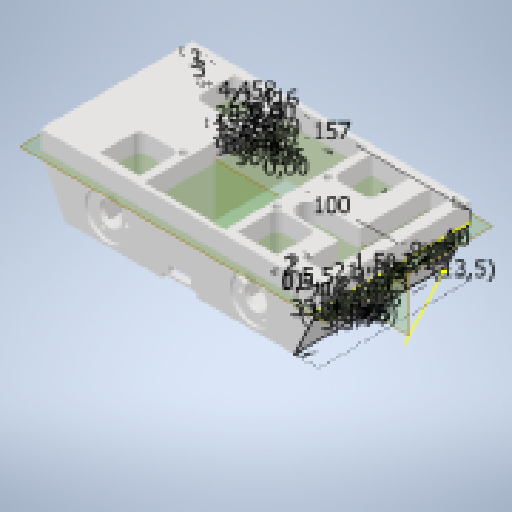
# Autodesk Inventor part: low_part
Saved by Autodesk Inventor 2025 (Build 290162000, 162)
## iProperties
Created: 2026-06-26
Part Number: low_part
Material: Типовые
Document SubType Name: Sheet Metal
Designer: garin
Density: 1 g/cm^3
Appearance: По умолчанию
Sheet Metal Rule: По умолчанию
Mass: 239.505 g
Surface Area: 434.405 cm^2
Volume: 239.505 cm^3
Author: garin
Autodesk Inventor part; units mm, degrees
ref_plane "YZ Plane" through (0, 0, 0) normal (1, 0, 0) x (0, 1, 0)
ref_plane "XZ Plane" through (0, 0, 0) normal (0, 1, 0) x (-1, 0, 0)
ref_plane "XY Plane" through (0, 0, 0) normal (0, 0, 1) x (1, 0, 0)
sketch "Эскиз2" plane through (0, 0, 0) normal (0, 0, 1) x (1, 0, 0)
  line L0 (0, 0) -> (-78.5, 0) construction
  line L1 (-78.5, 0) -> (78.5, 0)
  line L2 (0, 0) -> (-50, 0) construction
  line L3 (-50, 0) -> (-50, -28.5) construction
  line L4 (-50, -28.5) -> (-78.5, 0)
  line L5 (-50, -28.5) -> (50, -28.5)
  line L6 (50, -28.5) -> (78.5, 0)
  line L7 (-50, -28.5) -> (-45.542, -28.5) construction
  line L8 (-45.542, -28.5) -> (-45.542, -22.152) construction
  line L9 (-45.542, -22.152) -> (-50, -22.152) construction
  line L10 (-50, -22.152) -> (-50, -28.5) construction
  line L11 (-45.542, -22.152) -> (-45.542, -6.564) construction
  arc A0 (-45.542, -22.152) -> (-45.542, -6.564) centre (-50.0424, -14.358) ccw construction
  circle A1 centre (-45.542, -22.152) radius 1.3
  line L12 (-45.542, -22.152) -> (-32.0424, -14.358) construction
  line L13 (-45.542, -22.152) -> (-29.954, -22.152) construction
  circle A2 centre (-32.0424, -14.358) radius 1.3
  circle A3 centre (-45.542, -6.564) radius 1.3
  line L14 (-45.542, -6.564) -> (-32.0424, -14.358) construction
  circle A4 centre (-41.0424, -14.358) radius 12.5
  circle A5 centre (-41.0424, -14.358) radius 6.5
  line L15 (-41.0424, -14.358) -> (-41.0424, -26.858) construction
  line L16 (-41.0424, -14.358) -> (-34.7924, -25.1833) construction
  line L17 (-41.0424, -14.358) -> (-30.2171, -20.608) construction
  line L18 (-78.5, 0) -> (-75.5, 0) construction
  line L19 (-50, -28.5) -> (-47, -28.5) construction
  line L20 (-75.5, 0) -> (-47, -28.5)
  line L21 (-78.5, 0) -> (-75.5, 0) construction
  line L22 (-75.5, 0) -> (-75.5, -3) construction
  line L23 (-75.5, -3) -> (-78.5, -3) construction
  line L24 (-78.5, -3) -> (-78.5, 0) construction
  line L25 (-50, -28.5) -> (-50, -25.5) construction
  line L26 (-50, -28.5) -> (-47, -28.5) construction
  line L27 (-75.5, -3) -> (75.5, -3)
  line L28 (-75.5, -3) -> (75.5, -3) construction
  line L29 (0, 0) -> (0, -28.5) construction
  line L30 (75.5, 0) -> (47, -28.5)
  line L31 (-50, -25.5) -> (50, -25.5)
  line L32 (-50, -25.5) -> (50, -25.5) construction
  circle A6 centre (45.542, -22.152) radius 1.3
  circle A7 centre (32.0424, -14.358) radius 1.3
  circle A8 centre (45.542, -6.564) radius 1.3
  circle A9 centre (41.0424, -14.358) radius 12.5
  circle A10 centre (41.0424, -14.358) radius 6.5
  line L33 (41.0424, -14.358) -> (41.0424, -26.858) construction
  line L34 (41.0424, -14.358) -> (30.2171, -20.608) construction
  line L35 (-41.0424, -14.358) -> (-22.0786, -14.358) construction
  line L36 (-41.0424, -14.358) -> (-41.0424, -1.858)
  line L37 (-41.0424, -14.358) -> (-30.2171, -8.108)
  line L38 (41.0424, -14.358) -> (30.2171, -8.108)
  line L39 (41.0424, -14.358) -> (41.0424, -1.858)
  line L40 (-45.542, -6.564) -> (-50, -6.564) construction
  line L41 (-50, -6.564) -> (-50, 0) construction
  line L42 (-50, 0) -> (-45.542, 0) construction
  line L43 (-45.542, 0) -> (-45.542, -6.564) construction
  line L44 (-50, -25.5) -> (-27.584, -25.5)
  line L45 (-27.584, -25.5) -> (-27.584, 0)
  line L46 (-27.584, 0) -> (-50, 0)
  line L47 (-50, 0) -> (-50, -25.5)
  line L48 (27.584, -25.5) -> (27.584, 0)
  line L49 (50, 0) -> (50, -25.5)
  line L50 (-50, -28.5) -> (-65, -28.5)
  line L51 (-65, -28.5) -> (-78.5, 0)
  line L52 (-65, -28.5) -> (-62, -28.5)
  line L53 (-62, -28.5) -> (-75.5, 0)
  line L54 (-50, -25.5) -> (-63.4211, -25.5)
  line L55 (50, -28.5) -> (65, -28.5)
  line L56 (65, -28.5) -> (78.5, 0)
  line L57 (65, -28.5) -> (62, -28.5)
  line L58 (62, -28.5) -> (75.5, 0)
  point P0 (-72.5, -3)
  point P1 (72.5, -3)
  point P2 (-41.0424, -25.5)
  point P3 (-41.0424, -20.858)
  point P4 (-35.4132, -17.608)
  point P5 (-30.2171, -20.608)
  point P6 (-35.3762, -25.5)
  point P7 (35.3762, -25.5)
  point P8 (30.2171, -20.608)
  point P9 (35.4132, -17.608)
  point P10 (41.0424, -20.858)
  point P11 (41.0424, -25.5)
  point P12 (47, -28.5)
  point P13 (46.7086, -25.5)
  point P14 (41.0424, -26.858)
  point P15 (-46.7086, -25.5)
  point P16 (35.8226, -3)
  point P17 (41.0424, -3)
  point P18 (41.0424, -7.858)
  point P19 (35.4132, -11.108)
  point P20 (30.2171, -8.108)
  point P21 (-35.8226, -3)
  point P22 (-30.2171, -8.108)
  point P23 (-35.4132, -11.108)
  point P24 (-41.0424, -7.858)
  point P25 (-41.0424, -3)
  dimension "d0" = 78.5
  dimension "d1" = 157
  dimension "d2" = 50
  dimension "d3" = 28.5
  dimension "d4" = 100
  dimension "d15" = 4.458
  dimension "d16" = 6.348
  dimension "d17" = 15.588
  dimension "d18" = 9
  dimension "d19" = 2.6
  dimension "d20" = 15.588
  dimension "d21" = 30
  dimension "d22" = 2.6
  dimension "d23" = 2.6
  dimension "d24" = 25
  dimension "d25" = 13
  dimension "d26" = 12.5
  dimension "d29" = 30
  dimension "d31" = 3
  dimension "d32" = 3
  dimension "d33" = 3
  dimension "d34" = 90
  dimension "d35" = 0
  dimension "d36" = 0
  dimension "d48" = 4.458
  dimension "d49" = 22.416
  dimension "d151" = 15
  dimension "d152" = 3
  dimension "d153" = 15
  dimension "d154" = 3
  constraints: 118 end point, 17 symmetric about line, 13 point on line, 12 horizontal, 11 centre point, 9 parallel, 6 coincident, 5 perpendicular, 4 equal length, 3 point on circle, 3 vertical, 1 midpoint, 9 other
  measures "d0" distance of L0.start L0.end
  measures "d1" distance of L0.end L1.end
  measures "d2" distance of L0.start L2.end
  measures "d3" distance of L2.end L3.end
  measures "d4" distance of L3.end L5.end
  measures "d15" distance of L9.end L8.end
  measures "d16" distance of L8.end L7.end
  measures "d17" distance of L8.end L11.end
  measures "d18" radius of A0
  measures "d19" diameter of A1
  measures "d20" distance of L12.start L12.end
  measures "d21" angle of L13 L12
  measures "d22" diameter of A2
  measures "d23" diameter of A3
  measures "d24" diameter of A4
  measures "d25" diameter of A5
  measures "d26" distance of L15.start L15.end
  measures "d31" distance of L0.end L18.end
  measures "d32" distance of L3.end L19.end
  measures "d33" distance of L21.end L22.end
  measures "d34" angle of L26 L25
  measures "d35" distance between parallel lines of L27 L28
  measures "d36" distance between parallel lines of L31 L32
  measures "d48" distance of L41.end L42.end
  measures "d49" distance of L46.end L45.end
  measures "d151" distance of L3.end L50.end
  measures "d152" distance of L50.end L52.end
  measures "d153" distance of L5.end L55.end
  measures "d154" distance of L55.end L57.end
extrude "Выдавливание1" add sketch "Эскиз2" along normal blind 86 contours L1 L53 L27 L4 | L4 L53 L50 L51 | L1 L47 L27 L20 | L20 L27 L53 | L27 L53 L4 | L1 L45 L27 A4 L47 | L27 L47 A4 L20 | L20 L54 L4 L53 L27 | L4 L54 L53 | L53 L54 L4 L50 | L1 L48 L27 L45 | L27 A4 L47 | L31 A4 A9 L30 L5 L20 | L47 A4 L31 | L20 L5 L4 L54 | L1 L49 L27 A9 L48 | L45 L31 A4 L27 | L27 L48 L31 L45 | L27 L36 A5 L37 A4 L31 L47 | A4 L36 L27 | L47 A4 | L31 A4 | L1 L30 L27 L49 | L27 A9 L31 L48 | L27 L36 A4 | A4 L37 A5 L36 L27 | L30 L27 L58 L6 L5 | L58 L27 L30 | L1 L6 L27 L58 | L49 A9 L27 | L27 L30 L49 A9 | A9 L39 L27 | L27 L39 A10 L38 A9 | L36 L37 A5 | A5 L37 L36 | L6 L58 L55 | L31 A9 L49 | L56 L55 L58 L6 | L27 L6 L58 | A9 L49 L31 L38 A10 L39 L27 | L27 L39 A9 | A9 L49 | L31 A9 | L39 L38 A10 | A10 L38 L39 | A1 | A2 | A3 | A6 | A7 | A8
extrude "Выдавливание2" cut sketch "Эскиз2" along normal blind 5 contours A4 L37 A5 L36 L27 | L27 L39 A10 L38 A9 | L36 L37 A5 | A5 L37 L36 | L39 L38 A10 | A10 L38 L39 | A1 | A2 | A3 | A6 | A7 | A8
extrude "Выдавливание4" cut sketch "Эскиз2" along normal blind 2 contours L27 L36 A5 L37 A4 L31 L47 | A4 L36 L27 | L47 A4 | L31 A4 | L27 L36 A4 | A4 L37 A5 L36 L27 | A9 L39 L27 | L27 L39 A10 L38 A9 | L36 L37 A5 | A5 L37 L36 | A9 L49 L31 L38 A10 L39 L27 | L27 L39 A9 | A9 L49 | L31 A9 | L39 L38 A10 | A10 L38 L39 | A1 | A2 | A3 | A6 | A7 | A8
fillet "Сопряжение1" radius 2 4 edges at (35.4132, -11.108, 3.5) (41.0424, -7.858, 3.5) (-35.4132, -11.108, 3.5) (-41.0424, -7.858, 3.5)
extrude "Выдавливание6" cut sketch "Эскиз2" along normal blind 22.5 from surface at 5 contours L1 L45 L27 A4 L47 | L27 A4 L47 | L47 A4 L31 | L1 L49 L27 A9 L48 | L45 L31 A4 L27 | L27 L36 A5 L37 A4 L31 L47 | A4 L36 L27 | L27 A9 L31 L48 | L27 L36 A4 | A4 L37 A5 L36 L27 | L49 A9 L27 | A9 L39 L27 | L27 L39 A10 L38 A9 | L36 L37 A5 | A5 L37 L36 | L31 A9 L49 | A9 L49 L31 L38 A10 L39 L27 | L27 L39 A9 | L39 L38 A10 | A10 L38 L39 | A1 | A2 | A3 | A6 | A7 | A8
fillet "Сопряжение2" radius 4 4 edges at (50, -12.75, 27.5) (27.584, -12.75, 27.5) (-27.584, -12.75, 27.5) (-50, -12.75, 27.5)
ref_plane "РабПлоскость1" through (0, 0, 43) normal (0, 0, -1) x (-1, 0, 0)
mirror "Зеркальное отражение2" about plane through (0, 0, 43) normal (0, 0, -1) of "Выдавливание2", "Выдавливание6", "Сопряжение2", "Выдавливание4", "Сопряжение1"
sketch "Эскиз4" plane through (-78.5, 0, 0) normal (0, 1, 0) x (1, 0, 0)
  line L0 (78.5, 0) -> (78.5, -86) construction
  line L1 (28.5, -86) -> (128.5, -86) projected
  line L2 (0, 0) -> (0, -86) projected
  line L3 (0, -43) -> (157, -43) construction
  line L4 (157, 0) -> (157, -86) projected
  line L5 (78.5, -43) -> (101.4, -43) construction
  line L6 (101.4, -43) -> (101.4, -3) construction
  line L7 (101.4, -3) -> (78.5, -3) construction
  line L8 (78.5, -3) -> (78.5, -43) construction
  line L9 (101.4, -3) -> (55.6, -3)
  line L10 (55.6, -3) -> (55.6, -83)
  line L11 (55.6, -83) -> (101.4, -83)
  line L12 (101.4, -83) -> (101.4, -3)
  dimension "d53" = 22.9
  dimension "d54" = 40
  dimension "d55" = 45.8
  dimension "d56" = 80
  constraints: 20 end point, 4 midpoint, 4 parallel, 2 horizontal, 2 perpendicular
  measures "d53" distance of L7.end L6.end
  measures "d54" distance of L6.end L5.end
  measures "d55" distance of L11.end L10.end
  measures "d56" distance of L10.end L9.end
extrude "Выдавливание7" cut sketch "Эскиз4" against normal blind 28.5
sketch "Эскиз5" plane through (-78.5, 0, 0) normal (0, 1, 0) x (1, 0, 0)
  line L0 (0, 0) -> (157, 0)
  line L1 (157, 0) -> (157, -86)
  line L2 (157, -86) -> (0, -86)
  line L3 (0, -86) -> (0, 0)
  line L4 (55.6, -3) -> (101.4, -3) projected
  line L5 (55.6, -3) -> (55.6, -83) projected
  line L6 (101.4, -3) -> (55.6, -3)
  line L7 (55.6, -3) -> (55.6, -83)
  line L8 (55.6, -83) -> (101.4, -83)
  line L9 (101.4, -83) -> (101.4, -3)
  line L10 (104.4, 0) -> (52.6, 0)
  line L11 (52.6, 0) -> (52.6, -86)
  line L12 (52.6, -86) -> (104.4, -86)
  line L13 (104.4, -86) -> (104.4, 0)
  line L14 (3, -83) -> (154, -83)
  line L15 (154, -83) -> (154, -3)
  line L16 (154, -3) -> (3, -3)
  line L17 (3, -3) -> (3, -83)
  line L18 (104.4, 0) -> (106.084, 0)
  line L19 (106.084, 0) -> (106.084, -86)
  line L20 (106.084, -86) -> (104.4, -86)
  line L21 (104.4, -86) -> (104.4, 0)
  line L22 (52.6, 0) -> (50.916, 0)
  line L23 (50.916, 0) -> (50.916, -86)
  line L24 (50.916, -86) -> (52.6, -86)
  line L25 (52.6, -86) -> (52.6, 0)
  line L26 (50.916, 0) -> (52.916, 0) construction
  line L27 (0, -43) -> (157, -43) construction
  line L28 (78.5, -86) -> (78.5, 0) construction
  arc A0 (28.5, -23.5) -> (32.5, -27.5) centre (32.5, -23.5) ccw projected
  line L29 (46.916, -27.5) -> (32.5, -27.5) projected
  arc A1 (46.916, -27.5) -> (50.916, -23.5) centre (46.916, -23.5) ccw projected
  line L30 (50.916, -5) -> (50.916, -23.5) projected
  line L31 (50.916, -5) -> (28.5, -5) projected
  line L32 (28.5, -5) -> (28.5, -23.5) projected
  arc A2 (32.5, -58.5) -> (28.5, -62.5) centre (32.5, -62.5) ccw projected
  line L33 (28.5, -81) -> (28.5, -62.5) projected
  line L34 (50.916, -81) -> (28.5, -81) projected
  line L35 (50.916, -81) -> (50.916, -62.5) projected
  arc A3 (50.916, -62.5) -> (46.916, -58.5) centre (46.916, -62.5) ccw projected
  line L36 (46.916, -58.5) -> (32.5, -58.5) projected
  arc A4 (110.084, -58.5) -> (106.084, -62.5) centre (110.084, -62.5) ccw projected
  line L37 (106.084, -81) -> (106.084, -62.5) projected
  line L38 (128.5, -81) -> (106.084, -81) projected
  line L39 (128.5, -81) -> (128.5, -62.5) projected
  arc A5 (128.5, -62.5) -> (124.5, -58.5) centre (124.5, -62.5) ccw projected
  line L40 (124.5, -58.5) -> (110.084, -58.5) projected
  arc A6 (106.084, -23.5) -> (110.084, -27.5) centre (110.084, -23.5) ccw projected
  line L41 (124.5, -27.5) -> (110.084, -27.5) projected
  arc A7 (124.5, -27.5) -> (128.5, -23.5) centre (124.5, -23.5) ccw projected
  line L42 (128.5, -5) -> (128.5, -23.5) projected
  line L43 (128.5, -5) -> (106.084, -5) projected
  line L44 (106.084, -5) -> (106.084, -23.5) projected
  line L45 (46.916, -58.5) -> (55.6, -58.5) construction
  arc A8 (50.916, -62.5) -> (46.916, -58.5) centre (46.916, -62.5) ccw construction
  line L46 (46.916, -27.5) -> (55.6, -27.5) construction
  line L47 (55.6, -58.5) -> (52.1, -58.5) construction
  line L48 (52.1, -58.5) -> (52.1, -57.5) construction
  line L49 (52.1, -57.5) -> (55.6, -57.5) construction
  line L50 (55.6, -57.5) -> (55.6, -58.5) construction
  circle A9 centre (52.1, -57.5) radius 2.1
  circle A10 centre (52.1, -28.5) radius 2.1
  circle A11 centre (104.9, -57.5) radius 2.1
  circle A12 centre (104.9, -28.5) radius 2.1
  point P0 (50.916, -23.5)
  dimension "d59" = 157
  dimension "d60" = 86
  dimension "d61" = 3
  dimension "d62" = 3
  dimension "d63" = 1.684
  dimension "d64" = 1.684
  dimension "d72" = 3.5
  dimension "d73" = 1
  dimension "d74" = 4.2
  constraints: 66 end point, 14 parallel, 9 perpendicular, 6 horizontal, 4 centre point, 4 point on line, 3 midpoint, 3 symmetric about line, 3 tangent, 1 coincident, 1 vertical, 9 other
  measures "d59" distance of L1.end L2.end
  measures "d60" distance of L0.end L1.end
  measures "d61" distance between parallel lines of L9 L13
  measures "d62" distance between parallel lines of L2 L14
  measures "d63" distance of L19.end L20.end
  measures "d64" distance of L24.end L23.end
  measures "d72" distance of L48.end L49.end
  measures "d73" distance of L47.end L48.end
  measures "d74" diameter of A9
extrude "Выдавливание8" add sketch "Эскиз5" along normal blind 10.2 contours L0 L23 L16 L17 L14 L2 L3 | L0 L11 L16 L23 | L0 L13 L16 L4 L11 | L23 L31 L32 A0 L29 A1 A10 A9 A3 L36 A2 L33 L34 L14 L17 L16 | L16 L11 A10 L23 | L23 L14 L11 L2 | L0 L19 L16 L13 | L16 L5 L14 L11 A9 A10 | L11 L14 L8 L13 L2 | L23 A9 L11 L14 | L0 L1 L2 L19 L14 L15 L16 | L16 L19 A12 L13 | L13 A12 A11 L14 L9 L16 | L13 L14 L19 L2 | L16 L15 L14 L19 L38 L39 A5 L40 A4 A11 A12 A6 L41 A7 L42 L43 | L11 A9 L23 A10 | L13 A11 L19 L14 | A12 L19 A11 L13
sketch "Эскиз9" plane through (-65, -28.5, 0) normal (0, -1, 0) x (1, 0, 0)
  line L0 (130, 86) -> (143.5, 86) construction
  line L1 (0, 0) -> (130, 0) projected
  line L2 (143.5, 86) -> (130, 86) construction
  line L3 (130, 86) -> (130, 0) construction
  line L4 (130, 0) -> (143.5, 0) construction
  line L5 (143.5, 0) -> (143.5, 86) construction
  line L6 (130, 43) -> (87.9, 43) construction
  line L7 (87.9, 83) -> (87.9, 3) construction
  line L8 (130, 43) -> (87.9, 43) construction
  line L9 (87.9, 43) -> (87.9, 45) construction
  line L10 (87.9, 45) -> (130, 45) construction
  line L11 (130, 45) -> (130, 43) construction
  line L12 (130, 43) -> (87.9, 43) construction
  line L13 (87.9, 43) -> (87.9, 41) construction
  line L14 (87.9, 41) -> (130, 41) construction
  line L15 (130, 41) -> (130, 43) construction
  line L16 (130, 41) -> (127, 41) construction
  line L17 (127, 41) -> (106, 41)
  line L18 (106, 41) -> (106, 20)
  line L19 (106, 20) -> (127, 20)
  line L20 (127, 20) -> (127, 41)
  line L21 (127, 41) -> (124.364, 41) construction
  line L22 (124.364, 41) -> (124.364, 38.214) construction
  line L23 (124.364, 38.214) -> (127, 38.214) construction
  line L24 (127, 38.214) -> (127, 41) construction
  circle A0 centre (124.364, 38.214) radius 2
  line L25 (127, 41) -> (127, 45) construction
  line L26 (130, 45) -> (96.5, 45)
  line L27 (96.5, 45) -> (96.5, 56)
  line L28 (96.5, 56) -> (130, 56)
  line L29 (130, 56) -> (130, 45)
  line L30 (130, 45) -> (124.5, 45)
  line L31 (124.5, 45) -> (124.5, 56)
  line L32 (124.5, 56) -> (130, 56)
  line L33 (130, 56) -> (130, 45)
  line L34 (96.5, 56) -> (102, 56)
  line L35 (102, 56) -> (102, 45)
  line L36 (102, 45) -> (96.5, 45)
  line L37 (96.5, 45) -> (96.5, 56)
  arc A1 (124.5, 45) -> (124.5, 56) centre (124.5, 50.5) ccw
  arc A2 (102, 56) -> (102, 45) centre (102, 50.5) ccw
  circle A3 centre (102, 50.5) radius 2.1
  circle A4 centre (124.5, 50.5) radius 2.1
  line L38 (124.364, 38.214) -> (108.636, 38.214) construction
  circle A5 centre (108.636, 38.214) radius 2
  line L39 (124.5, 50.5) -> (117.5, 50.5) construction
  line L40 (124.5, 50.5) -> (131.5, 50.5) construction
  line L41 (102, 50.5) -> (109, 50.5) construction
  circle A6 centre (117.5, 50.5) radius 3
  circle A7 centre (109, 50.5) radius 3
  circle A8 centre (117.5, 50.5) radius 3.5 construction
  line L42 (122.4, 50.5) -> (121, 50.5) construction
  line L43 (121.7, 50.5) -> (121.7, 45)
  line L44 (121.7, 50.5) -> (121.7, 56)
  line L45 (113.25, 45) -> (113.25, 56) construction
  line L46 (104.8, 50.5) -> (104.8, 45)
  line L47 (104.8, 50.5) -> (104.8, 56)
  arc A9 (124.5, 44.5) -> (124.5, 56.5) centre (124.5, 50.5) ccw
  arc A10 (102, 56.5) -> (102, 44.5) centre (102, 50.5) ccw
  line L48 (124.5, 56.5) -> (102, 56.5)
  line L49 (124.5, 44.5) -> (102, 44.5)
  line L50 (121.7, 45) -> (121.7, 44.5)
  line L51 (121.7, 56) -> (121.7, 56.5)
  line L52 (104.8, 56) -> (104.8, 56.5)
  line L53 (104.8, 45) -> (104.8, 44.5)
  line L54 (106, 20) -> (107.5, 20)
  line L55 (107.5, 20) -> (125.5, 20)
  line L56 (125.5, 20) -> (125.5, 23)
  line L57 (125.5, 23) -> (107.5, 23)
  line L58 (107.5, 23) -> (107.5, 20)
  point P0 (65, 0)
  dimension "d173" = 4.2
  dimension "d181" = 7
  dimension "d155" = 13.5
  dimension "d156" = 86
  dimension "d157" = 2
  dimension "d158" = 2
  dimension "d159" = 3
  dimension "d160" = 21
  dimension "d161" = 21
  dimension "d162" = 2.636
  dimension "d163" = 2.786
  dimension "d164" = 4
  dimension "d168" = 33.5
  dimension "d169" = 11
  dimension "d170" = 5.5
  dimension "d171" = 5.5
  dimension "d172" = 4.2
  dimension "d174" = 15.728
  dimension "d175" = 4
  dimension "d176" = 7
  dimension "d177" = 180
  dimension "d178" = 7
  dimension "d179" = 6
  dimension "d180" = 6
  dimension "d182" = 0.5
  dimension "d183" = 0.5
  dimension "d196" = 1.5
  dimension "d197" = 18
  dimension "d198" = 3
  constraints: 112 end point, 19 parallel, 19 point on line, 13 horizontal, 13 perpendicular, 9 centre point, 8 point on circle, 7 coincident, 6 midpoint, 6 tangent, 3 symmetric about line, 2 horizontal alignment, 1 collinear, 4 other
  measures "d155" distance of L4.end L1.end
  measures "d156" distance of L1.end L2.end
  measures "d157" distance of L8.end L9.end
  measures "d158" distance of L13.end L12.end
  measures "d159" distance of L14.end L16.end
  measures "d160" distance of L19.end L18.end
  measures "d161" distance of L18.end L17.end
  measures "d162" distance of L23.end L22.end
  measures "d163" distance of L22.end L21.end
  measures "d164" diameter of A0
  measures "d168" distance of L27.end L28.end
  measures "d169" distance of L26.end L27.end
  measures "d170" distance of L31.end L32.end
  measures "d171" distance of L35.end L36.end
  measures "d172" diameter of A3
  measures "d174" distance of L38.start L38.end
  measures "d175" diameter of A5
  measures "d176" distance of L39.start L39.end
  measures "d177" angle of L39 L40
  measures "d178" distance of L41.start L41.end
  measures "d179" diameter of A6
  measures "d180" diameter of A7
  measures "d182" radial gap between concentric circles of A1 A9
  measures "d183" radial gap between concentric circles of A2 A10
  measures "d196" distance of L18.end L54.end
  measures "d197" distance of L57.end L56.end
  measures "d198" distance of L56.end L55.end
extrude "Выдавливание17" cut sketch "Эскиз9" along normal blind 30 from surface at -38.7 contours L26 A9 L49 L50 | A1 L29 A9 L26 | L26 L43 L44 L28 L31 A4 | L31 A4 A1 | L50 L49 L53 L26 | L26 L46 L47 L28 L44 L43 | A4 L31 | L31 A4 | A1 L28 A9 L29 | L29 A9 | L53 L49 A10 L26 | L26 L35 A3 L28 L47 L46 | L28 L51 L48 A9 | A2 L35 A3 | L26 A10 L27 A2 | L28 L52 L48 L51 | A3 L35 | L35 A3 | L27 A10 | L27 A10 L28 A2 | L28 A10 L48 L52 | A6 | A7
extrude "Выдавливание18" cut sketch "Эскиз9" along normal blind 2 from surface at -8.7 contours L50 L49 L53 L26 | L26 L46 L47 L28 L44 L43 | L28 L52 L48 L51 | A6 | A7
extrude "Выдавливание19" cut sketch "Эскиз9" along normal blind 8.7 from surface at -8.7 contours A6 | A7
extrude "Выдавливание20" cut sketch "Эскиз9" along normal blind 6.7 from surface at -8.7 contours A4 L31 | L31 A4 | A3 L35 | L35 A3
extrude "Выдавливание21" cut sketch "Эскиз9" against normal blind 1.5 contours L20 L19 L56 L57 L58 L18 L17 | L19 L58 L57 L56 | A0 | A5
extrude "Выдавливание22" cut sketch "Эскиз9" against normal blind 6 from surface at -1.5 contours A0 | A5
extrude "Выдавливание23" cut sketch "Эскиз9" against normal blind 6 contours L19 L58 L57 L56
sketch "Эскиз10" plane through (65, -28.5, 86) normal (0.9037378, -0.4280863, 0) x (0, 0, -1)
  line L0 (86, 31.5357) -> (0, 31.5357) projected
  line L1 (86, -55.6512) -> (86, 0) projected
  line L2 (0, 31.5357) -> (86, 31.5357)
  line L3 (86, 31.5357) -> (86, 0)
  line L4 (86, 0) -> (0, 0)
  line L5 (0, 0) -> (0, 31.5357)
  line L6 (43, 31.5357) -> (43, 0) construction
  line L7 (11, 28.0357) -> (73, 28.0357)
  line L8 (73, 28.0357) -> (73, 19.0357)
  line L9 (73, 19.0357) -> (11, 19.0357)
  line L10 (11, 19.0357) -> (11, 28.0357)
  line L11 (42, 28.0357) -> (42, 19.0357)
  line L12 (11, 19.0357) -> (12.8, 19.0357) construction
  line L13 (12.8, 19.0357) -> (12.8, 21.5357) construction
  line L14 (12.8, 21.5357) -> (11, 21.5357) construction
  line L15 (11, 21.5357) -> (11, 19.0357) construction
  circle A0 centre (12.8, 21.5357) radius 1.75
  line L16 (12.8, 21.5357) -> (12.8, 25.5357) construction
  circle A1 centre (12.8, 25.5357) radius 1.75
  line L17 (73, 19.0357) -> (63.25, 19.0357) construction
  line L18 (63.25, 19.0357) -> (63.25, 21.1357) construction
  line L19 (63.25, 21.1357) -> (73, 21.1357) construction
  line L20 (73, 21.1357) -> (73, 19.0357) construction
  circle A2 centre (63.25, 21.1357) radius 1.75
  line L21 (11, 28.0357) -> (38.5, 28.0357) construction
  line L22 (38.5, 28.0357) -> (47.5, 28.0357) construction
  line L23 (47.5, 28.0357) -> (47.5, 19.0357)
  line L24 (47.5, 19.0357) -> (38.5, 19.0357) construction
  line L25 (38.5, 19.0357) -> (38.5, 28.0357)
  line L26 (73.5, 28.5357) -> (10.5, 28.5357)
  line L27 (10.5, 28.5357) -> (10.5, 18.5357)
  line L28 (10.5, 18.5357) -> (73.5, 18.5357)
  line L29 (73.5, 18.5357) -> (73.5, 28.5357)
  line L30 (47.5, 28.0357) -> (48, 28.0357) construction
  line L31 (48, 28.0357) -> (48, 28.5357) construction
  line L32 (48, 28.5357) -> (47.5, 28.5357) construction
  line L33 (47.5, 28.5357) -> (47.5, 28.0357) construction
  line L34 (48, 28.5357) -> (48, 18.5357)
  line L35 (43, 28.0357) -> (43, 19.0357) construction
  line L36 (38, 28.5357) -> (38, 18.5357)
  line L37 (43, 28.5357) -> (43, 28.0357) construction
  line L38 (43, 31.5357) -> (43, 28.5357) construction
  line L39 (73.5, 28.5357) -> (81.5, 28.5357)
  line L40 (81.5, 28.5357) -> (81.5, 18.5357)
  line L41 (81.5, 18.5357) -> (73.5, 18.5357)
  line L42 (73.5, 18.5357) -> (73.5, 28.5357)
  line L43 (73.5, 28.5357) -> (67.5, 28.5357)
  line L44 (67.5, 28.5357) -> (67.5, 18.5357)
  line L45 (67.5, 18.5357) -> (73.5, 18.5357)
  line L46 (73.5, 18.5357) -> (73.5, 28.5357)
  point P0 (86, -2.0691)
  point P1 (43, 23.5357)
  point P2 (38, 28.5357)
  point P3 (38, 18.5357)
  point P4 (73.5, 18.5357)
  point P5 (73.5, 18.5357)
  dimension "d201" = 86
  dimension "d202" = 62
  dimension "d203" = 9
  dimension "d206" = 1.8
  dimension "d207" = 2.5
  dimension "d208" = 3.5
  dimension "d209" = 4
  dimension "d210" = 3.5
  dimension "d211" = 9.75
  dimension "d212" = 2.1
  dimension "d213" = 3.5
  dimension "d214" = 27.5
  dimension "d215" = 9
  dimension "d216" = 9
  dimension "d217" = 0.5
  dimension "d218" = 0.5
  dimension "d219" = 3
  dimension "d220" = 8
  dimension "d221" = 10
  dimension "d231" = 6
  constraints: 90 end point, 18 parallel, 11 perpendicular, 8 horizontal, 7 midpoint, 6 point on line, 3 centre point, 3 coincident, 2 symmetric about line, 1 vertical, 3 other
  measures "d201" distance of L1.end L4.end
  measures "d202" distance of L8.end L9.end
  measures "d203" distance of L7.end L8.end
  measures "d206" distance of L14.end L13.end
  measures "d207" distance of L13.end L12.end
  measures "d208" diameter of A0
  measures "d209" distance of L16.start L16.end
  measures "d210" diameter of A1
  measures "d211" distance of L18.end L19.end
  measures "d212" distance of L17.end L18.end
  measures "d213" diameter of A2
  measures "d214" distance of L7.start L21.end
  measures "d215" distance of L23.end L24.end
  measures "d216" distance of L22.end L23.end
  measures "d217" distance between parallel lines of L7 L26
  measures "d218" distance of L32.end L31.end
  measures "d219" distance of L6.start L37.start
  measures "d220" distance of L40.end L41.end
  measures "d221" distance of L39.end L40.end
  measures "d231" distance of L45.end L44.end
extrude "Выдавливание24" cut sketch "Эскиз10" against normal blind 6 contours L7 L36 L26 L34 | L25 L9 L36 L7 | L7 L11 L9 L25 | L7 L23 L9 L11 | L9 L34 L28 L36 | L7 L34 L9 L23
extrude "Выдавливание25" cut sketch "Эскиз10" against normal blind 10.2 from surface at -6 contours L7 L36 L26 L34 | L25 L9 L36 L7 | L7 L11 L9 L25 | L7 L23 L9 L11 | L36 L9 L10 L7 | L7 L10 L9 L36 L28 L27 L26 | L9 L34 L28 L36 | L7 L34 L9 L23 | L34 L26 L44 L7 | L7 L44 L9 L34 | L44 L26 L29 L28 L9 L8 L7 | L7 L8 L9 L44 | L9 L44 L28 L34 | L39 L40 L41 L29 | A0 | A1 | A2
ref_plane "РабПлоскость4" through (71.7933, -0.1427, 48) normal (0, -1, 0) x (1, 0, 0)
sketch "Эскиз12" plane through (71.7933, -0.1427, 48) normal (0, -1, 0) x (1, 0, 0)
  line L0 (0, 27.5) -> (-4.2809, 27.5) projected
  line L1 (-13.499, -43.5) -> (-4.2809, -43.5) projected
  line L2 (0, 27.5) -> (-13.499, 27.5)
  line L3 (-13.499, 27.5) -> (-13.499, -43.5)
  line L4 (-13.499, -43.5) -> (0, -43.5)
  line L5 (0, -43.5) -> (0, 27.5)
  line L6 (-13.499, -43.5) -> (-11.286, -43.5)
  line L7 (-11.286, -43.5) -> (-11.286, 27.5)
  line L8 (-11.286, 27.5) -> (-13.499, 27.5)
  line L9 (-13.499, 27.5) -> (-13.499, -43.5)
  point P0 (-71.7933, -48)
  point P1 (-11.286, -43.5)
  dimension "d228" = 2.213
  constraints: 16 end point, 4 parallel, 2 horizontal, 2 perpendicular, 1 point on line
  measures "d228" distance of L8.end L7.end
extrude "Выдавливание26" cut sketch "Эскиз12" against normal blind 12 from surface at 0 contours L5 L4 L1 L7 L2 L0
extrude "Выдавливание27" cut sketch "Эскиз10" along normal blind 5 from surface at -6 contours A0 | A1 | A2
extrude "Выдавливание28" cut sketch "Эскиз10" along normal blind 5 from surface at -6 contours L44 L26 L29 L28 L9 L8 L7 | L7 L8 L9 L44 | L39 L40 L41 L29
sketch "Эскиз13" plane through (0, 0, 0) normal (0, 0, -1) x (-1, 0, 0)
  line L0 (0, 0) -> (0, -28.5) construction
  line L1 (-22.9, -28.5) -> (22.9, -28.5) construction
  line L2 (-10, -28.5) -> (10, -28.5)
  line L3 (10, -28.5) -> (10, -26)
  line L4 (10, -26) -> (-10, -26)
  line L5 (-10, -26) -> (-10, -28.5)
  line L6 (-6.4, -24.5) -> (6.4, -24.5)
  line L7 (6.4, -24.5) -> (6.4, -20.5)
  line L8 (6.4, -20.5) -> (-6.4, -20.5)
  line L9 (-6.4, -20.5) -> (-6.4, -24.5)
  line L10 (-10, -28.5) -> (10, -28.5) construction
  line L11 (10, -28.5) -> (10, -24.5) construction
  line L12 (10, -24.5) -> (-10, -24.5) construction
  line L13 (-10, -24.5) -> (-10, -28.5) construction
  line L14 (0, -20.5) -> (0, -24.5) construction
  dimension "d234" = 20
  dimension "d235" = 2.5
  dimension "d240" = 12.8
  dimension "d241" = 4
  dimension "d242" = 20
  dimension "d243" = 4
  constraints: 28 end point, 6 parallel, 5 midpoint, 3 horizontal, 3 perpendicular
  measures "d234" distance of L4.end L3.end
  measures "d235" distance of L3.end L2.end
  measures "d240" distance of L8.end L7.end
  measures "d241" distance of L7.end L6.end
  measures "d242" distance of L12.end L11.end
  measures "d243" distance of L11.end L10.end
extrude "Выдавливание29" cut sketch "Эскиз13" against normal blind 3
extrude "Выдавливание30" cut sketch "Эскиз13" along normal blind 3 from surface at -86
sketch "Эскиз14" plane through (-22.9, -28.5, 83) normal (1, 0, 0) x (0, 0, -1)
  circle A0 centre (58.6346, 61.3723) radius 4
  arc A1 (45.4346, 65.8723) -> (45.4346, 56.8723) centre (45.4346, 61.3723) ccw
  line L0 (45.4346, 56.8723) -> (59.9346, 56.8723)
  arc A2 (59.9346, 56.8723) -> (59.9346, 65.8723) centre (59.9346, 61.3723) ccw
  line L1 (59.9346, 65.8723) -> (45.4346, 65.8723)
  line L2 (38.1846, 61.8473) -> (40.9597, 61.8473)
  line L3 (38.1846, 60.8973) -> (38.1846, 61.8473)
  line L4 (40.9597, 60.8973) -> (38.1846, 60.8973)
  arc A3 (40.9597, 61.8473) -> (40.9597, 60.8973) centre (45.4346, 61.3723) ccw
  line L5 (64.4094, 60.8973) -> (67.1846, 60.8973)
  line L6 (67.1846, 60.8973) -> (67.1846, 61.8473)
  line L7 (67.1846, 61.8473) -> (64.4094, 61.8473)
  arc A4 (64.4094, 60.8973) -> (64.4094, 61.8473) centre (59.9346, 61.3723) ccw
  line L8 (83, 38.7) -> (-3, 38.7) projected
  line L9 (-3, 38.7) -> (83, 38.7)
  line L10 (83, 38.7) -> (83, 0)
  line L11 (83, 0) -> (-3, 0)
  line L12 (-3, 0) -> (-3, 38.7)
  line L13 (40, 38.7) -> (40, 0) construction
  line L14 (40, 0) -> (40, 3) construction
  line L15 (32.75, 12) -> (47.25, 12)
  line L16 (47.25, 12) -> (47.25, 3)
  line L17 (47.25, 3) -> (32.75, 3)
  line L18 (32.75, 3) -> (32.75, 12)
  arc A5 (32.75, 12) -> (32.75, 3) centre (32.75, 7.5) ccw
  arc A6 (47.25, 3) -> (47.25, 12) centre (47.25, 7.5) ccw
  line L19 (30.5769, 66.2028) -> (33.3519, 66.2028)
  line L20 (33.3519, 66.2028) -> (33.3519, 65.2528)
  line L21 (33.3519, 65.2528) -> (30.5769, 65.2528)
  line L22 (30.5769, 65.2528) -> (30.5769, 66.2028)
  line L23 (33.3519, 65.7278) -> (33.3269, 65.7278)
  point P0 (83, 28.5)
  point P1 (52.6846, 61.3723)
  dimension "d244" = 3
  dimension "d245" = 14.5
  dimension "d246" = 9
  dimension "d247" = 2.775
  dimension "d248" = 0.95
  dimension "d249" = 0.025
  constraints: 46 end point, 12 point on circle, 7 centre point, 6 midpoint, 6 parallel, 4 horizontal, 3 perpendicular, 1 point on line
  measures "d244" distance of L14.end L13.end
  measures "d245" distance of L16.end L17.end
  measures "d246" distance of L15.end L16.end
  measures "d247" distance of L20.end L21.end
  measures "d248" distance of L19.end L20.end
  measures "d249" distance of L23.start L23.end
